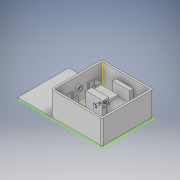
# Autodesk Inventor part: ohisje
Saved by Autodesk Inventor 2019 (Build 230136000, 136)
## iProperties
Created: 2020-07-23
Part Number: ohisje
Material: Generic
Document SubType Name: Modeling
Designer: lukad
Density: 1 g/cm^3
Appearance: Default
Author: lukad
Autodesk Inventor part; units mm, degrees
ref_plane "YZ Plane" through (0, 0, 0) normal (1, 0, 0) x (0, 1, 0)
ref_plane "XZ Plane" through (0, 0, 0) normal (0, 1, 0) x (-1, 0, 0)
ref_plane "XY Plane" through (0, 0, 0) normal (0, 0, 1) x (1, 0, 0)
sketch "Sketch1" plane through (0, 0, 0) normal (0, 1, 0) x (-1, 0, 0)
  line L0 (17.7167, 30.9206) -> (-32.2833, 30.9206)
  line L1 (-32.2833, 30.9206) -> (-32.2833, -19.0794)
  line L2 (-32.2833, -19.0794) -> (17.7167, -19.0794)
  line L3 (17.7167, -19.0794) -> (17.7167, 30.9206)
  line L4 (19.7167, 32.9206) -> (-34.2833, 32.9206)
  line L5 (-34.2833, 32.9206) -> (-34.2833, -21.0794)
  line L6 (-34.2833, -21.0794) -> (19.7167, -21.0794)
  line L7 (19.7167, -21.0794) -> (19.7167, 32.9206)
  line L8 (19.7167, 32.9206) -> (54.7167, 32.9206)
  line L9 (54.7167, 32.9206) -> (54.7167, -21.0794)
  line L10 (54.7167, -21.0794) -> (19.7167, -21.0794)
  line L11 (19.7167, -21.0794) -> (19.7167, 32.9206)
  point P0 (0, 0)
  dimension "d0" = 50
  dimension "d1" = 50
  dimension "d2" = 2
  dimension "d3" = 2
  dimension "d4" = 2
  dimension "d5" = 2
  dimension "d6" = 35
  dimension "d7" = 54
  constraints: 24 end point, 6 parallel, 3 horizontal, 3 perpendicular
  measures "d0" distance of L2.end L0.start
  measures "d1" distance of L1.end L2.end
  measures "d2" distance between parallel lines of L6 L2
  measures "d3" distance between parallel lines of L4 L0
  measures "d4" distance between parallel lines of L7 L3
  measures "d5" distance between parallel lines of L1 L5
  measures "d6" distance of L9.end L10.end
  measures "d7" distance of L8.end L9.end
extrude "Extrusion1" add sketch "Sketch1" along normal blind 27 contours L7 L6 L5 L4
sketch "Sketch2" plane through (34.2833, 0, 32.9206) normal (1, 0, 0) x (0, 0, -1)
  line L0 (0, 0) -> (0, 27) projected
  line L1 (54, 0) -> (54, 27) projected
  line L2 (0, 0) -> (54, 0)
  line L3 (54, 0) -> (54, 2)
  line L4 (54, 2) -> (0, 2)
  line L5 (0, 2) -> (0, 0)
  point P0 (32.9206, 0)
  dimension "d10" = 2
  constraints: 8 end point, 2 parallel, 1 horizontal, 1 perpendicular, 1 point on line
  measures "d10" distance between parallel lines of L2 L4
extrude "Extrusion2" add sketch "Sketch2" against normal blind 89
fillet "Fillet1" radius 2 7 edges at (34.2833, 13.5, 32.9206) (34.2833, 13.5, -21.0794) (-19.7167, 14.5, -21.0794) (-19.7167, 14.5, 32.9206) (34.2833, 0, 5.9206) (-10.2167, 0, 32.9206) (-10.2167, 0, -21.0794)
sketch "Sketch3" plane through (-17.7167, 2, 30.9206) normal (0, 1, 0) x (1, 0, 0)
  line L0 (9, 9) -> (1, 9)
  line L1 (1, 9) -> (1, 17)
  line L2 (1, 17) -> (9, 17)
  line L3 (9, 17) -> (9, 9)
  line L4 (50, 0) -> (0, 0) projected
  line L5 (0, 0) -> (0, 50) projected
  line L6 (8.05, 9.95) -> (1.95, 9.95)
  line L7 (1.95, 9.95) -> (1.95, 16.05)
  line L8 (1.95, 16.05) -> (8.05, 16.05)
  line L9 (8.05, 16.05) -> (8.05, 9.95)
  line L10 (0, 25) -> (50, 25)
  line L11 (0, 50) -> (50, 50) projected
  line L12 (50, 50) -> (50, 0) projected
  line L13 (9, 41) -> (1, 41)
  line L14 (1, 41) -> (1, 33)
  line L15 (1, 33) -> (9, 33)
  line L16 (9, 33) -> (9, 41)
  line L17 (8.05, 40.05) -> (1.95, 40.05)
  line L18 (1.95, 40.05) -> (1.95, 33.95)
  line L19 (1.95, 33.95) -> (8.05, 33.95)
  line L20 (8.05, 33.95) -> (8.05, 40.05)
  line L21 (36, 25) -> (18, 25)
  line L22 (18, 25) -> (18, 47)
  line L23 (18, 47) -> (36, 47)
  line L24 (36, 47) -> (36, 25)
  line L25 (36, 25) -> (18, 25)
  line L26 (18, 25) -> (18, 15)
  line L27 (18, 15) -> (36, 15)
  line L28 (36, 15) -> (36, 25)
  line L29 (36, 47) -> (18, 47)
  line L30 (18, 47) -> (18, 43)
  line L31 (18, 43) -> (36, 43)
  line L32 (36, 43) -> (36, 47)
  line L33 (36, 15) -> (34, 15)
  line L34 (34, 15) -> (34, 47)
  line L35 (34, 47) -> (36, 47)
  line L36 (36, 47) -> (36, 15)
  line L37 (34, 21) -> (33, 21)
  line L38 (33, 21) -> (33, 22)
  line L39 (33, 22) -> (34, 22)
  line L40 (34, 22) -> (34, 21)
  line L41 (34, 28) -> (33, 28)
  line L42 (33, 28) -> (33, 29)
  line L43 (33, 29) -> (34, 29)
  line L44 (34, 29) -> (34, 28)
  line L45 (34, 39) -> (33, 39)
  line L46 (33, 39) -> (33, 40)
  line L47 (33, 40) -> (34, 40)
  line L48 (34, 40) -> (34, 39)
  point P0 (17.7167, 30.9206)
  dimension "d26" = 9
  dimension "d27" = 8
  dimension "d28" = 1
  dimension "d29" = 6.1
  dimension "d30" = 0.95
  dimension "d31" = 0.95
  dimension "d33" = 25
  dimension "d34" = 25
  dimension "d39" = 16
  dimension "d74" = 22
  dimension "d75" = 18
  dimension "d76" = 18
  dimension "d77" = 10
  dimension "d78" = 18
  dimension "d87" = 4
  dimension "d90" = 2
  dimension "d93" = 6
  dimension "d94" = 1
  dimension "d95" = 1
  dimension "d96" = 3
  dimension "d97" = 3
  dimension "d98" = 1
  dimension "d99" = 1
  dimension "d100" = 10
  dimension "d101" = 1
  dimension "d102" = 1
  constraints: 90 end point, 18 parallel, 13 perpendicular, 9 horizontal, 8 symmetric about line, 6 point on line, 1 midpoint
  measures "d26" distance between parallel lines of L4 L0
  measures "d27" distance between parallel lines of L0 L2
  measures "d28" distance between parallel lines of L5 L1
  measures "d29" distance between parallel lines of L8 L6
  measures "d30" distance between parallel lines of L3 L9
  measures "d31" distance between parallel lines of L8 L2
  measures "d33" distance between parallel lines of L4 L10
  measures "d34" distance between parallel lines of L11 L10
  measures "d39" distance between parallel lines of L2 L15
  measures "d74" distance between parallel lines of L21 L23
  measures "d75" distance of L26.end L27.end
  measures "d76" distance of L22.end L23.end
  measures "d77" distance of L27.end L21.start
  measures "d78" distance between parallel lines of L5 L22
  measures "d87" distance between parallel lines of L23 L31
  measures "d90" distance between parallel lines of L34 L36
  measures "d93" distance between parallel lines of L27 L37
  measures "d94" distance between parallel lines of L34 L38
  measures "d95" distance between parallel lines of L37 L39
  measures "d96" distance between parallel lines of L10 L39
  measures "d97" distance between parallel lines of L41 L10
  measures "d98" distance between parallel lines of L43 L41
  measures "d99" distance of L41.start L41.end
  measures "d100" distance between parallel lines of L45 L43
  measures "d101" distance between parallel lines of L34 L46
  measures "d102" distance between parallel lines of L47 L45
extrude "Extrusion3" add sketch "Sketch3" along normal blind 15 contours L0 L1 L2 L3
sketch "Sketch4" plane through (-17.7167, 2, 30.9206) normal (0, 1, 0) x (1, 0, 0)
  point P0 (17.7167, 30.9206)
extrude "Extrusion4" add sketch "Sketch3" along normal blind 15 contours L16 L15 L14 L13
fillet "Fillet2" radius 1 8 edges at (-8.7167, 9.5, -2.0794) (-8.7167, 9.5, -10.0794) (-16.7167, 9.5, -2.0794) (-16.7167, 9.5, -10.0794) (-8.7167, 9.5, 13.9206) (-8.7167, 9.5, 21.9206) (-16.7167, 9.5, 21.9206) (-16.7167, 9.5, 13.9206)
sketch "Sketch5" plane through (-17.7167, 27, 30.9206) normal (1, 0, 0) x (0, 0, -1)
  circle A0 centre (25, -11) radius 1.8
  line L0 (50, -25) -> (50, 0) projected
  line L1 (0, -25) -> (50, -25) projected
  point P0 (30.9206, -27)
  dimension "d41" = 3.6
  dimension "d42" = 25
  dimension "d43" = 14
  constraints: 1 centre point
  measures "d41" diameter of A0
  measures "d42" distance from line of L0 A0.centre
  measures "d43" distance from line of L1 A0.centre
extrude "Extrusion5" cut sketch "Sketch5" against normal blind 1
sketch "Sketch6" plane through (-17.7167, 2, 30.9206) normal (0, 1, 0) x (1, 0, 0)
  line L0 (10.5, 9.0139) -> (13.5, 9.0139)
  line L1 (13.5, 9.0139) -> (13.5, 41.0139)
  line L2 (13.5, 41.0139) -> (10.5, 41.0139)
  line L3 (10.5, 41.0139) -> (10.5, 9.0139)
  line L4 (2, 9) -> (8, 9) projected
  line L5 (8, 41) -> (2, 41) projected
  line L6 (9, 16) -> (9, 10) projected
  point P0 (17.7167, 30.9206)
  dimension "d46" = 3
  dimension "d47" = 32
  dimension "d48" = 1.5
  constraints: 8 end point, 4 parallel, 1 horizontal, 1 perpendicular
  measures "d46" distance between parallel lines of L1 L3
  measures "d47" distance between parallel lines of L2 L0
  measures "d48" distance between parallel lines of L6 L3
extrude "Extrusion6" [suppressed]
sketch "Sketch7" plane through (-4.2167, 2, 21.9067) normal (1, 0, 0) x (0, 0, -1)
  circle A0 centre (15.9861, 14) radius 1.8
  circle A1 centre (15.9861, 14) radius 1.8 projected
  point P0 (21.9067, -2)
  dimension "d51" = 3.6
  constraints: 1 centre point, 1 concentric
  measures "d51" diameter of A0
extrude "Extrusion7" [suppressed]
sketch "Sketch8" plane through (-4.2167, 2, 21.9067) normal (1, 0, 0) x (0, 0, -1)
  line L0 (32.0428, 14) -> (0, 14)
  line L1 (0, 0) -> (0, 14) projected
  line L2 (0, 14) -> (32, 14) projected
  line L3 (32, 0) -> (0, 0) projected
  point P0 (21.9067, -2)
  dimension "d54" = 14
  constraints: 2 end point, 1 collinear, 1 point on line
  measures "d54" distance between parallel lines of L3 L0
sketch "Sketch9" plane through (-17.7167, 27, 30.9206) normal (1, 0, 0) x (0, 0, -1)
  line L0 (3.6476, -12) -> (44.1553, -12)
  line L1 (44.1553, -12) -> (44.1553, -24)
  line L2 (44.1553, -24) -> (3.6476, -24)
  line L3 (3.6476, -24) -> (3.6476, -12)
  line L4 (0, -25) -> (50, -25) projected
  point P0 (30.9206, -27)
  dimension "d55" = 12
  dimension "d56" = 1
  constraints: 8 end point, 2 parallel, 1 horizontal, 1 perpendicular
  measures "d55" distance between parallel lines of L2 L0
  measures "d56" distance between parallel lines of L4 L2
extrude "Extrusion8" [suppressed]
sketch "Sketch10" plane through (-17.7167, 17, 30.9206) normal (0, 1, 0) x (1, 0, 0)
  line L0 (8.05, 16.05) -> (1.95, 16.05) projected
  line L1 (2, 17) -> (8, 17) projected
  line L2 (2.9, 16.05) -> (7.1, 16.05)
  line L3 (7.1, 16.05) -> (7.1, 17)
  line L4 (7.1, 17) -> (2.9, 17)
  line L5 (2.9, 17) -> (2.9, 16.05)
  line L6 (1.95, 9.95) -> (1.95, 16.05) projected
  line L7 (8.05, 16.05) -> (8.05, 9.95) projected
  point P0 (17.7167, 30.9206)
  dimension "d59" = 0.95
  dimension "d60" = 0.95
  constraints: 8 end point, 2 parallel, 2 point on line, 1 horizontal, 1 perpendicular
  measures "d59" distance between parallel lines of L6 L5
  measures "d60" distance between parallel lines of L7 L3
extrude "Extrusion9" cut sketch "Sketch10" against normal blind 10
sketch "Sketch11" plane through (-17.7167, 17, 30.9206) normal (0, 1, 0) x (1, 0, 0)
  line L0 (8, 33) -> (2, 33) projected
  line L1 (8.05, 33.95) -> (1.95, 33.95) projected
  line L2 (2.9, 33) -> (7.1, 33)
  line L3 (7.1, 33) -> (7.1, 33.95)
  line L4 (7.1, 33.95) -> (2.9, 33.95)
  line L5 (2.9, 33.95) -> (2.9, 33)
  line L6 (1.95, 33.95) -> (1.95, 40.05) projected
  line L7 (8.05, 40.05) -> (8.05, 33.95) projected
  point P0 (17.7167, 30.9206)
  dimension "d63" = 0.95
  dimension "d64" = 0.95
  dimension "d65" = 0.95
  constraints: 8 end point, 2 parallel, 2 point on line, 1 horizontal, 1 perpendicular
  measures "d63" distance between parallel lines of L6 L5
  measures "d64" distance between parallel lines of L7 L3
  measures "d65" distance between parallel lines of L1 L0
extrude "Extrusion10" cut sketch "Sketch11" against normal blind 10
sketch "Sketch12" plane through (-17.7167, 27, 30.9206) normal (1, 0, 0) x (0, 0, -1)
  circle A0 centre (25, -11) radius 3
  circle A1 centre (25, -11) radius 1.8 projected
  point P0 (30.9206, -27)
  dimension "d68" = 6
  constraints: 1 centre point, 1 concentric
  measures "d68" diameter of A0
extrude "Extrusion11" add sketch "Sketch12" along normal blind 2
sketch "Sketch13" plane through (-17.7167, 16, 30.9206) normal (0, 1, 0) x (1, 0, 0)
  line L0 (13.5, 41.0139) -> (13.5, 9.0139) projected
  line L1 (13.5, 41.0139) -> (10.5, 41.0139) projected
  line L2 (13.5, 31.0139) -> (10.5, 31.0139)
  line L3 (10.5, 31.0139) -> (10.5, 41.0139)
  line L4 (10.5, 41.0139) -> (13.5, 41.0139)
  line L5 (13.5, 41.0139) -> (13.5, 31.0139)
  line L6 (10.5, 9.0139) -> (13.5, 9.0139) projected
  point P0 (17.7167, 30.9206)
  dimension "d71" = 10
  constraints: 8 end point, 3 parallel, 1 horizontal, 1 perpendicular, 1 point on line
  measures "d71" distance between parallel lines of L1 L2
extrude "Extrusion12" [suppressed]
sketch "Sketch14" plane through (-17.7167, 2, 30.9206) normal (0, 1, 0) x (1, 0, 0)
  point P0 (17.7167, 30.9206)
extrude "Extrusion13" add sketch "Sketch3" along normal blind 9 contours L28 L27 L34 L10 | L10 L34 L31 L24 | L22 L31 L34 L47 L46 L45 L43 L42 L41 L10 | L10 L34 L39 L38 L37 L27 L26 | L31 L34 L23 L24 | L22 L23 L34 L31 | L34 L37 L38 L39 | L41 L42 L43 L34 | L34 L45 L46 L47
sketch "Sketch15" plane through (-17.7167, 11, 30.9206) normal (0, 1, 0) x (1, 0, 0)
  line L0 (36, 47) -> (36, 15) projected
  line L1 (18, 47) -> (18, 15) projected
  line L2 (36, 15) -> (18, 15)
  line L3 (18, 15) -> (18, 19)
  line L4 (18, 19) -> (36, 19)
  line L5 (36, 19) -> (36, 15)
  point P0 (17.7167, 30.9206)
  dimension "d81" = 4
  constraints: 8 end point, 2 parallel, 1 horizontal, 1 perpendicular, 1 point on line
  measures "d81" distance between parallel lines of L4 L2
extrude "Extrusion14" add sketch "Sketch15" along normal blind 16
extrude "Extrusion16" add sketch "Sketch3" along normal blind 20 contours L31 L34 L23 L24 | L22 L23 L34 L31
extrude "Extrusion17" [suppressed]
extrude "Extrusion18" [suppressed]
extrude "Extrusion19" [suppressed]
extrude "Extrusion20" [suppressed]
sketch "Sketch17" plane through (18.2833, 11, 11.9206) normal (0, 0, -1) x (-1, 0, 0)
  line L0 (0, -9) -> (0, 16) projected
  line L1 (18, -9) -> (18, 16) projected
  line L2 (0, 16) -> (18, 16)
  line L3 (18, 16) -> (18, 11)
  line L4 (18, 11) -> (0, 11)
  line L5 (0, 11) -> (0, 16)
  point P0 (18.2833, -11)
  dimension "d109" = 5
  constraints: 8 end point, 2 parallel, 1 horizontal, 1 perpendicular, 1 point on line
  measures "d109" distance between parallel lines of L2 L4
extrude "Extrusion21" add sketch "Sketch17" along normal blind 12
sketch "Sketch18" plane through (-17.7167, 11, 30.9206) normal (0, 1, 0) x (1, 0, 0)
  line L0 (18, 19) -> (36, 19) projected
  line L1 (27, 19) -> (24, 19)
  line L2 (24, 19) -> (24, 23)
  line L3 (24, 23) -> (27, 23)
  line L4 (27, 23) -> (27, 19)
  line L5 (18, 43) -> (18, 19) projected
  line L6 (24, 26.8826) -> (27, 26.8826)
  line L7 (27, 26.8826) -> (27, 30.8826)
  line L8 (27, 30.8826) -> (24, 30.8826)
  line L9 (24, 30.8826) -> (24, 26.8826)
  line L10 (24, 26.8826) -> (27, 26.8826)
  line L11 (27, 26.8826) -> (27, 23)
  line L12 (27, 23) -> (24, 23)
  line L13 (24, 23) -> (24, 26.8826)
  point P0 (17.7167, 30.9206)
  dimension "d112" = 9
  dimension "d113" = 3
  dimension "d114" = 4
  dimension "d115" = 3
  dimension "d116" = 4
  constraints: 24 end point, 6 parallel, 3 horizontal, 3 perpendicular, 1 midpoint
  measures "d112" distance between parallel lines of L5 L4
  measures "d113" distance of L2.end L3.end
  measures "d114" distance between parallel lines of L3 L0
  measures "d115" distance of L6.start L6.end
  measures "d116" distance of L8.end L6.start
sketch "Sketch19" plane through (-17.7167, 11, 30.9206) normal (0, 1, 0) x (1, 0, 0)
  point P0 (17.7167, 30.9206)
extrude "Extrusion22" add sketch "Sketch18" along normal blind 10 contours L2 L3 L4 L0 | L9 L8 L7 L6
extrude "Extrusion23" add sketch "Sketch18" along normal blind 3 contours L13 L6 L11 L3
sketch "Sketch20" plane through (9.2833, 21, 7.9206) normal (0, 0, -1) x (-1, 0, 0)
  point P0 (9.2833, -21)
sketch "Sketch21" plane through (9.2833, 21, 7.9206) normal (0, 0, -1) x (-1, 0, 0)
  line L0 (0, 0) -> (3, 0) projected
  line L1 (0, 0) -> (3, 0)
  line L2 (3, 0) -> (3, -3)
  line L3 (3, -3) -> (0, -3)
  line L4 (0, -3) -> (0, 0)
  point P0 (9.2833, -21)
  dimension "d121" = 3
  constraints: 8 end point, 2 parallel, 1 horizontal, 1 perpendicular
  measures "d121" distance between parallel lines of L0 L3
extrude "Extrusion24" add sketch "Sketch21" along normal blind 4
sketch "Sketch22" plane through (18.2833, 2, 15.9206) normal (1, 0, 0) x (0, 0, -1)
  line L0 (5.5, 7) -> (26.5, 7)
  line L1 (26.5, 7) -> (26.5, 0)
  line L2 (26.5, 0) -> (5.5, 0)
  line L3 (5.5, 0) -> (5.5, 7)
  line L4 (4, 9) -> (28, 9) projected
  line L5 (28, 9) -> (28, 20) projected
  point P0 (15.9206, -2)
  dimension "d124" = 2
  dimension "d125" = 7
  dimension "d126" = 21
  dimension "d129" = 1.5
  constraints: 8 end point, 2 parallel, 1 horizontal, 1 perpendicular
  measures "d124" distance between parallel lines of L4 L0
  measures "d125" distance between parallel lines of L2 L0
  measures "d126" distance between parallel lines of L1 L3
  measures "d129" distance between parallel lines of L5 L1
extrude "Extrusion25" cut sketch "Sketch22" against normal blind 20
sketch "Sketch23" plane through (18.2833, 11, -0.0794) normal (0, 0, -1) x (-1, 0, 0)
  line L0 (18, 16) -> (0, 16) projected
  line L1 (0, 16) -> (0, 11) projected
  line L2 (18, 16) -> (0, 16)
  line L3 (0, 16) -> (0, 13.5)
  line L4 (0, 13.5) -> (18, 13.5)
  line L5 (18, 13.5) -> (18, 16)
  point P0 (18.2833, -11)
  dimension "d130" = 2.5
  constraints: 8 end point, 2 parallel, 1 horizontal, 1 midpoint, 1 perpendicular
  measures "d130" distance between parallel lines of L4 L0
extrude "Extrusion26" cut sketch "Sketch23" against normal blind 10
equation "\"d1\" = d0"
equation "\"d76\" = d75"
equation "\"d98\" = d95"
equation "\"d99\" = d94"
equation "\"d101\" = d99"
equation "\"d102\" = d95"
equation "\"d54\" = d43"
equation "\"d115\" = d113"
equation "\"d116\" = d114"
body "Solid1"
